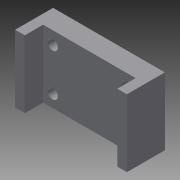
# Autodesk Inventor part: hd16_standoff
Saved by Autodesk Inventor 2014 (Build 180170000, 170)
## iProperties
Created: 2014-10-03
Part Number: hd16_standoff
Material: Generic
Document SubType Name: Modeling
Designer: Matthew
Density: 1 g/cm^3
Appearance: Default
Author: Matthew
Autodesk Inventor part; units mm, degrees
ref_plane "YZ Plane" through (0, 0, 0) normal (1, 0, 0) x (0, 1, 0)
ref_plane "XZ Plane" through (0, 0, 0) normal (0, 1, 0) x (-1, 0, 0)
ref_plane "XY Plane" through (0, 0, 0) normal (0, 0, 1) x (1, 0, 0)
sketch "Sketch1" plane through (0, 0, 0) normal (0, 1, 0) x (-1, 0, 0)
  line L0 (29, -17.5) -> (-29, -17.5)
  line L1 (-29, -17.5) -> (-29, 17.5)
  line L2 (-29, 17.5) -> (29, 17.5)
  line L3 (29, 17.5) -> (29, -17.5)
  line L4 (29, -17.5) -> (-29, 17.5) construction
  line L5 (-29, -17.5) -> (29, 17.5) construction
  point P0 (0, 0)
  dimension "d0" = 58
  dimension "d1" = 35
  constraints: 12 end point, 2 midpoint, 2 parallel, 1 horizontal, 1 perpendicular
  measures "d0" distance of L1.end L2.end
  measures "d1" distance of L0.end L1.end
extrude "Extrusion1" add sketch "Sketch1" along normal blind 10.16
sketch "Sketch2" plane through (0, 0, 0) normal (0, -1, 0) x (1, 0, 0)
  line L0 (-29, -17.5) -> (29, -17.5) projected
  line L1 (29, -17.5) -> (29, 17.5) projected
  line L2 (29, 17.5) -> (-29, 17.5) projected
  line L3 (-29, 17.5) -> (-29, -17.5) projected
  line L4 (-24, 17.5) -> (-24, -17.5)
  line L5 (24, 17.5) -> (24, -17.5)
  point P0 (0, 0)
  dimension "d4" = 5
  dimension "d5" = 5
  constraints: 4 end point, 4 point on line, 2 perpendicular
  measures "d4" distance between parallel lines of L1 L5
  measures "d5" distance between parallel lines of L3 L4
extrude "Extrusion2" add sketch "Sketch2" along normal blind 9.525 contours L3 L2 L4 L0 | L5 L2 L1 L0
sketch "Sketch3" plane through (0, 10.16, 0) normal (0, 1, 0) x (1, 0, 0)
  line L0 (29, 17.5) -> (-29, 17.5) projected
  line L1 (-29, 17.5) -> (-29, -17.5) projected
  point P0 (0, 0)
  point P1 (-19, 11)
  point P2 (19, 11)
  point P3 (-19, -11)
  point P4 (19, -11)
  dimension "d10" = 38
  dimension "d13" = 22
  dimension "d16" = 10
  dimension "d17" = 58
  dimension "d18" = 35
  dimension "d19" = 6.5
  constraints: 1 horizontal, 1 vertical, 3 other
  measures "d10" distance of point (-19, 11) point (19, 11)
  measures "d13" distance of point (-19, 11) point (-19, -11)
  measures "d16" distance from line of L1 point (-19, 11)
  measures "d17" distance of L0.start L0.end
  measures "d18" distance of L0.end L1.end
  measures "d19" distance from line of L0 point (-19, 11)
hole "Hole1" at (-19, 10.16, -11) at (19, 10.16, -11) at (-19, 10.16, 11) at (19, 10.16, 11) direction (0, -1, 0) diameter 5.25 end through all
equation "\"d5\" = d4"
equation "\"d16\" = -0.5 * d10 + 0.5 * d17"
equation "\"d19\" = -0.5 * d13 + 0.5 * d18"
body "Solid1"
